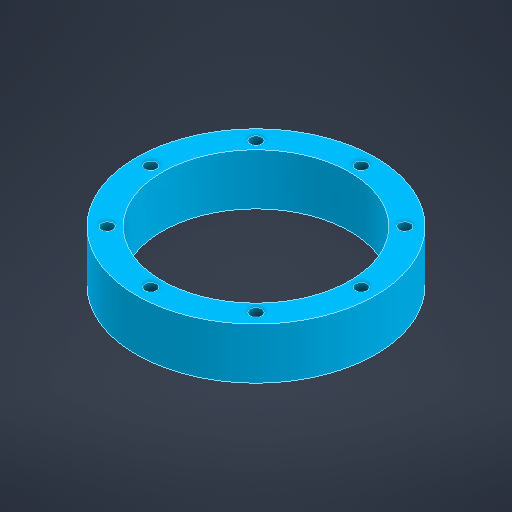
# Autodesk Inventor part: Gearbox_MainBody
Saved by Autodesk Inventor 2025 (Build 290162000, 162)
## iProperties
Created: 2024-01-31
Part Number: Gearbox_MainBody
Material: Generic
Document SubType Name: Modeling
Designer: avsar
Density: 1 g/cm^3
Appearance: Sky Blue Medium
Author: avsar
Autodesk Inventor part; units mm, degrees
ref_plane "YZ Plane" through (0, 0, 0) normal (1, 0, 0) x (0, 1, 0)
ref_plane "XZ Plane" through (0, 0, 0) normal (0, 1, 0) x (-1, 0, 0)
ref_plane "XY Plane" through (0, 0, 0) normal (0, 0, 1) x (1, 0, 0)
sketch "Sketch1" plane through (0, 0, 0) normal (0, 1, 0) x (-1, 0, 0)
  circle A0 centre (0, 0) radius 33
  circle A1 centre (0, 0) radius 42
  dimension "d0" = 66
  dimension "d1" = 84
  constraints: 2 centre point, 2 coincident
  measures "d0" diameter of A0
  measures "d1" diameter of A1
extrude "Extrusion1" add sketch "Sketch1" along normal blind 18
sketch "Sketch2" plane through (0, 18, 0) normal (0, 1, 0) x (1, 0, 0)
  circle A0 centre (0, 37) radius 2
  circle A1 centre (-26.163, 26.163) radius 2
  circle A2 centre (-37, 0) radius 2
  circle A3 centre (-26.163, -26.163) radius 2
  circle A4 centre (0, -37) radius 2
  circle A5 centre (26.163, -26.163) radius 2
  circle A6 centre (37, 0) radius 2
  circle A7 centre (26.163, 26.163) radius 2
  point P0 (0, 0)
  dimension "d4" = 4
  dimension "d5" = 37
  dimension "d8" = 360
  constraints: 8 centre point, 1 vertical alignment, 17 other
  measures "d4" diameter of A0
  measures "d5" distance of point (0, 0) A0.centre
extrude "Extrusion2" cut sketch "Sketch2" against normal up to surface (18 mm away)
body "Solid1"
